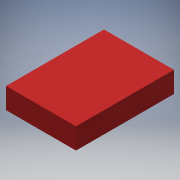
# Autodesk Inventor part: CardDeck
Saved by Autodesk Inventor 2017 SP1 (Build 210196100, 196)
## iProperties
Created: 2016-10-19
Part Number: CardDeck
Material: ABS Plastic
Document SubType Name: Modeling
Designer: steele
Density: 1.06 g/cm^3
Appearance: Light Red
Author: steele
Autodesk Inventor part; units mm, degrees
ref_plane "YZ Plane" through (0, 0, 0) normal (1, 0, 0) x (0, 1, 0)
ref_plane "XZ Plane" through (0, 0, 0) normal (0, 1, 0) x (-1, 0, 0)
ref_plane "XY Plane" through (0, 0, 0) normal (0, 0, 1) x (1, 0, 0)
sketch "Sketch1" plane through (0, 0, 0) normal (0, 1, 0) x (-1, 0, 0)
  line L0 (31.75, 44.45) -> (-31.75, 44.45)
  line L1 (-31.75, 44.45) -> (-31.75, -44.45)
  line L2 (-31.75, -44.45) -> (31.75, -44.45)
  line L3 (31.75, -44.45) -> (31.75, 44.45)
  line L4 (31.75, 44.45) -> (-31.75, -44.45) construction
  line L5 (-31.75, 44.45) -> (31.75, -44.45) construction
  point P0 (0, 0)
  dimension "d0" = 63.5
  dimension "d1" = 88.9
  constraints: 12 end point, 2 midpoint, 2 parallel, 1 horizontal, 1 perpendicular
  measures "d0" distance of L1.end L2.end
  measures "d1" distance of L2.end L0.start
extrude "Extrusion1" add sketch "Sketch1" along normal blind 19.05
equation "\"d0\" = cardDeckWidth"
equation "\"d1\" = cardDeckLength"
equation "\"d2\" = cardDeckDepth"
equation "\"cardDeckWidth\" = 63.5"
equation "\"cardDeckLength\" = 88.9"
equation "\"cardDeckDepth\" = 19.05"
body "Solid1"
